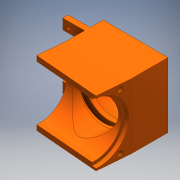
# Autodesk Inventor part: Trappe lancement
Saved by Autodesk Inventor 2016 SP1 (Build 200210100, 210)
## iProperties
Created: 2017-04-26
Part Number: Trappe lancement
Material: Plastique ABS
Document SubType Name: Modeling
Designer: dimercur
Density: 1.06 g/cm^3
Appearance: Lisse - Orange clair
Mass: 75.5193 g
Surface Area: 203.785 cm^2
Volume: 71.2446 cm^3
Author: dimercur
Autodesk Inventor part; units mm, degrees
ref_plane "YZ Plane" through (0, 0, 0) normal (1, 0, 0) x (0, 1, 0)
ref_plane "XZ Plane" through (0, 0, 0) normal (0, 1, 0) x (-1, 0, 0)
sketch "Esquisse13" plane through (0, 0, 0) normal (0, 1, 0) x (-1, 0, 0)
  line L0 (0, 0) -> (-60, 0)
  line L1 (-60, 0) -> (-60, -60)
  line L2 (-60, -60) -> (0, -60)
  line L3 (0, -60) -> (0, 0)
  dimension "d54" = 60
  dimension "d55" = 60
  constraints: 8 end point, 2 parallel, 1 horizontal, 1 perpendicular
  measures "d54" distance between parallel lines of L2 L0
  measures "d55" distance of L0.start L0.end
extrude "Extrusion11" add sketch "Esquisse13" along normal blind 34
sketch "Esquisse14" plane through (0, 34, 0) normal (0, 1, 0) x (1, 0, 0)
  circle A0 centre (30, 30) radius 23
  line L0 (0, 0) -> (60, 0) projected
  line L1 (60, 0) -> (60, 60) projected
  dimension "d58" = 30
  dimension "d59" = 30
  dimension "d60" = 46
  constraints: 1 centre point
  measures "d58" distance from line of L0 A0.centre
  measures "d59" distance from line of L1 A0.centre
  measures "d60" diameter of A0
extrude "Extrusion12" cut sketch "Esquisse14" against normal through all
sketch "Esquisse15" plane through (0, 34, 0) normal (0, 1, 0) x (1, 0, 0)
  circle A0 centre (30, 30) radius 25.25
  circle A1 centre (30, 30) radius 23 projected
  point P0 (0, 0)
  dimension "d63" = 50.5
  constraints: 1 centre point, 1 concentric
  measures "d63" diameter of A0
extrude "Extrusion13" cut sketch "Esquisse15" against normal blind 20
sketch "Esquisse16" plane through (0, 0, -60) normal (-1, 0, 0) x (0, 0, 1)
  line L0 (0, 0) -> (60, 0) projected
  line L1 (0, 0) -> (0, 34) projected
  line L2 (0, 9.5) -> (48, 9.5)
  line L3 (48, 9.5) -> (48, 5)
  line L4 (48, 5) -> (0, 5)
  line L5 (0, 5) -> (0, 9.5)
  dimension "d69" = 48
  dimension "d70" = 5
  dimension "d71" = 4.5
  constraints: 8 end point, 2 parallel, 1 horizontal, 1 perpendicular, 1 point on line
  measures "d69" distance of L2.start L2.end
  measures "d70" distance between parallel lines of L0 L4
  measures "d71" distance of L2.end L3.end
extrude "Extrusion14" cut sketch "Esquisse16" against normal blind 43
ref_plane "Plan de construction5" through (0, 5, -60) normal (0.0830455, 0.9965458, 0) x (0, 0, 1)
sketch "Esquisse18" plane through (0, 5, -60) normal (0.0830455, 0.9965458, 0) x (0, 0, 1)
  line L0 (0, 57.3844) -> (0, -2.4083) projected
  line L1 (60, 60.208) -> (0, 60.208) projected
  line L2 (0, 0.4152) -> (60, 0.4152)
  line L3 (60, 0.4152) -> (60, 60.208)
  line L4 (60, 60.208) -> (0, 60.208)
  line L5 (0, 60.208) -> (0, 0.4152)
  point P0 (60, 0.4152)
  constraints: 8 end point, 2 parallel, 1 horizontal, 1 perpendicular, 1 point on line
extrude "Extrusion15" add sketch "Esquisse18" against normal blind 30
sketch "Esquisse19" plane through (-2.4914, -24.8964, -60) normal (-0.0830455, -0.9965458, 0) x (0.9965458, -0.0830455, 0)
  circle A0 centre (30.104, 30) radius 23
  ellipse E0 centre (30.104, 30) end of major axis (7.0243, 30) minor radius 23 projected
  point P0 (0.4152, 60)
  dimension "d76" = 46
  constraints: 1 centre point, 2 other
  measures "d76" diameter of A0
extrude "Extrusion16" cut sketch "Esquisse19" against normal blind 30 contours A0
sketch "Esquisse20" plane through (0, 0, -60) normal (-0.9965458, 0.0830455, 0) x (0, 0, 1)
  line L0 (53, -25.0173) -> (7, -25.0173) projected
  circle A0 centre (30, -25.0173) radius 25.25
  line L1 (0, 0) -> (0, -25.0173) projected
  point P0 (60, 0)
  dimension "d79" = 50.5
  dimension "d80" = 30
  constraints: 1 centre point, 1 midpoint
  measures "d79" diameter of A0
  measures "d80" distance from line of A0.centre L1
extrude "Extrusion17" cut sketch "Esquisse20" against normal through all
sketch "Esquisse21" plane through (60, 0, 0) normal (0.9965458, -0.0830455, 0) x (0, 0, -1)
  circle A0 centre (30, -30) radius 28
  arc A1 (55.25, -30) -> (4.75, -30) centre (30, -30) ccw projected
  point P0 (0, -4.9827)
  dimension "d83" = 56
  constraints: 1 centre point, 1 concentric
  measures "d83" diameter of A0
extrude "Extrusion18" cut sketch "Esquisse21" against normal blind 4
sketch "Esquisse22" plane through (0, 34, -60) normal (-1, 0, 0) x (0, 0, 1)
  line L0 (0, -17) -> (9.5, -17)
  line L1 (9.5, -17) -> (9.5, -12)
  line L2 (9.5, -12) -> (0, -12)
  line L3 (0, -12) -> (0, -17)
  line L4 (60, -34) -> (60, 0) projected
  line L5 (60, -17) -> (50.5, -17)
  line L6 (50.5, -17) -> (50.5, -12)
  line L7 (50.5, -12) -> (60, -12)
  line L8 (60, -12) -> (60, -17)
  line L9 (0, -24.5) -> (48, -24.5) projected
  dimension "d86" = 5
  dimension "d88" = 41
  dimension "d92" = 7.5
  dimension "d93" = 60
  dimension "d94" = 9.5
  constraints: 16 end point, 4 parallel, 2 horizontal, 2 perpendicular, 2 point on line, 1 midpoint
  measures "d86" distance between parallel lines of L2 L0
  measures "d88" distance between parallel lines of L6 L1
  measures "d92" distance between parallel lines of L9 L0
  measures "d93" distance between parallel lines of L4 L3
  measures "d94" distance of L1.end L2.end
extrude "Extrusion19" add sketch "Esquisse22" along normal blind 20
sketch "Esquisse24" plane through (0, 22, 0) normal (0, 1, 0) x (1, 0, 0)
  circle A0 centre (-15, 5.75) radius 1.5
  circle A1 centre (-5, 5.75) radius 1.5
  circle A2 centre (-5, 54.25) radius 1.5
  circle A3 centre (-15, 54.25) radius 1.5
  line L0 (0, 0) -> (-20, 0) projected
  line L1 (0, 50.5) -> (-20, 50.5) projected
  line L2 (0, 60) -> (0, 0) projected
  dimension "d95" = 3
  dimension "d97" = 48.5
  dimension "d98" = 48.5
  dimension "d99" = 10
  dimension "d100" = 10
  dimension "d101" = 3.75
  dimension "d102" = 3.75
  dimension "d103" = 5
  dimension "d104" = 5
  constraints: 4 centre point, 3 equal radius
  measures "d95" diameter of A0
  measures "d97" distance of A3.centre A0.centre
  measures "d98" distance of A1.centre A2.centre
  measures "d99" distance of A1.centre A0.centre
  measures "d100" distance of A2.centre A3.centre
  measures "d101" distance from line of A3.centre L1
  measures "d102" distance from line of L1 A2.centre
  measures "d103" distance from line of L2 A2.centre
  measures "d104" distance from line of L2 A1.centre
extrude "Extrusion20" cut sketch "Esquisse24" against normal through all
sketch "Esquisse25" plane through (0, 0, -26.5797) normal (-0.9965458, 0.0830455, 0) x (0, 0, 1)
  circle A0 centre (-28.9203, -4.5) radius 2.25
  circle A1 centre (22.0797, -4.5) radius 2.25
  line L0 (-33.4203, 0) -> (-33.4203, -25.0173) projected
  line L1 (26.5797, 0) -> (26.5797, -25.0173) projected
  line L2 (0, 0) -> (26.5797, 0) projected
  line L3 (-33.4203, 0) -> (-6.8407, 0) projected
  dimension "d107" = 4.5
  dimension "d108" = 4.5
  dimension "d109" = 4.5
  dimension "d110" = 4.5
  dimension "d111" = 4.5
  constraints: 2 centre point, 1 equal radius
  measures "d107" diameter of A0
  measures "d108" distance from line of A0.centre L0
  measures "d109" distance from line of L1 A1.centre
  measures "d110" distance from line of L2 A1.centre
  measures "d111" distance from line of L3 A0.centre
extrude "Extrusion21" cut sketch "Esquisse25" against normal through all
equation "\"d94\" = -0.5 * d88 + 0.5 * d93"
equation "\"d98\" = d97"
equation "\"d100\" = d99"
equation "\"d102\" = d101"
equation "\"d104\" = d103"
equation "\"d109\" = d108"
equation "\"d111\" = d110"
